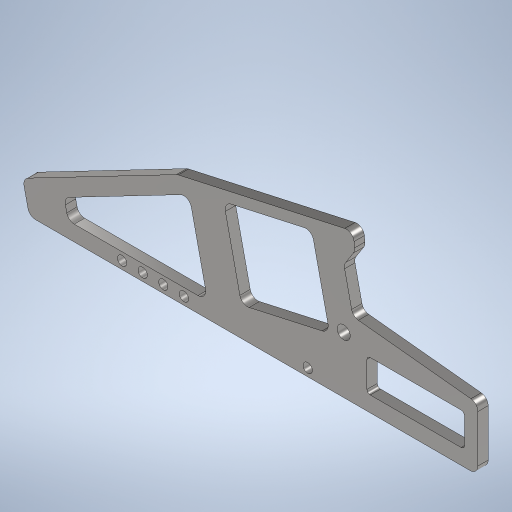
# Autodesk Inventor part: Uprights
Saved by Autodesk Inventor 2023.4 (Build 274418000, 418)
## iProperties
Created: 2024-02-11
Part Number: Uprights
Material: Stainless Steel
Document SubType Name: Modeling
Designer: Nathan Cai
Density: 8 g/cm^3
Appearance: Semi-Polished
Mass: 70.807 g
Surface Area: 79.2126 cm^2
Volume: 8.85087 cm^3
Author: Nathan Cai
Autodesk Inventor part; units mm, degrees
ref_plane "YZ Plane" through (0, 0, 0) normal (1, 0, 0) x (0, 1, 0)
ref_plane "XZ Plane" through (0, 0, 0) normal (0, 1, 0) x (-1, 0, 0)
ref_plane "XY Plane" through (0, 0, 0) normal (0, 0, 1) x (1, 0, 0)
sketch "Sketch1" plane through (0, 0, 0) normal (0, 0, 1) x (1, 0, 0)
  line L0 (0, 0) -> (0, 136.2362)
  line L1 (-14.9636, 12.2907) -> (-39.7615, 17.7883)
  line L2 (-39.7615, 17.7883) -> (-33.7485, 44.911)
  line L3 (-33.7485, 44.911) -> (-8.9506, 39.4135)
  line L4 (-8.9506, 39.4135) -> (-14.9636, 12.2907)
  line L5 (-39.7615, 17.7883) -> (-8.9506, 39.4135) construction
  line L6 (-33.7485, 44.911) -> (-14.9636, 12.2907) construction
  circle A0 centre (-57.15, 12.7) radius 3.3401
  circle A1 centre (-57.15, 12.7) radius 6.35
  line L7 (0, 0) -> (-57.847, 6.3884)
  line L8 (-62.7825, 15.6321) -> (0, 136.2362)
  line L9 (-21.3496, 42.1622) -> (-27.3626, 15.0395) construction
  line L10 (0, 104.775) -> (-14.6831, 108.0302)
  line L11 (-35.4518, 7.8896) -> (-23.0529, 5.1408)
  line L12 (-23.0529, 5.1408) -> (-24.4273, -1.0586) construction
  line L13 (-24.4273, -1.0586) -> (-36.8262, 1.6901) construction
  line L14 (-36.8262, 1.6901) -> (-35.4518, 7.8896) construction
  line L15 (-35.4518, 7.8896) -> (-40.7688, 4.5023)
  line L16 (-8.9506, 39.4135) -> (-33.7485, 44.911)
  line L17 (-56.4271, 15.9609) -> (-57.15, 12.7) construction
  line L18 (-57.15, 12.7) -> (-60.4109, 13.4229) construction
  line L19 (-29.2523, 6.5152) -> (-36.1243, -24.4822) construction
  line L20 (-56.356, 15.9443) -> (-9.0672, 106.7852)
  line L21 (-35.1857, 56.612) -> (0, 48.8115)
  line L22 (-4.7625, 49.8673) -> (-4.7625, 105.8308)
  line L23 (-30.3721, 55.5448) -> (-10.3247, 94.0556)
  line L24 (-10.3247, 94.0556) -> (-4.7625, 92.8225)
  circle A2 centre (-17.3978, 7.9523) radius 2
  line L25 (0, 13.4938) -> (-4.7625, 13.4937) construction
  line L26 (-4.7625, 13.4937) -> (-4.7625, 24.6063) construction
  line L27 (-4.7625, 24.6063) -> (0, 24.6063) construction
  line L28 (0, 24.6063) -> (0, 13.4938) construction
  line L29 (-4.7625, 19.05) -> (0, 19.05) construction
  circle A3 centre (-2.3812, 19.05) radius 1.4224
  line L30 (-4.7625, 57.15) -> (0, 57.15) construction
  circle A4 centre (-2.3813, 57.15) radius 1.4224
  circle A5 centre (-2.3813, 63.5) radius 1.4224
  circle A6 centre (-2.3813, 69.85) radius 1.4224
  circle A7 centre (-2.3813, 76.2) radius 1.4224
  line L31 (-22.792, 92.4532) -> (-17.8635, 89.8876)
  circle A8 centre (-57.15, 12.7) radius 9.525 construction
  line L32 (-14.7625, 0.7937) -> (-4.7625, 0.7938)
  line L33 (-4.7625, 0.7938) -> (-4.7625, -29.2062)
  line L34 (-4.7625, -29.2062) -> (-14.7625, -29.2062)
  line L35 (-14.7625, -29.2062) -> (-14.7625, 0.7937)
  line L36 (-14.7625, 0.7937) -> (-4.7625, -29.2062) construction
  line L37 (-4.7625, 0.7938) -> (-14.7625, -29.2062) construction
  line L38 (-19.05, -33.3375) -> (0, -33.3375)
  line L39 (0, -33.3375) -> (0, 0)
  line L40 (-23.0529, 5.1408) -> (-19.05, -33.3375)
  circle A9 centre (-17.3978, 7.9523) radius 6.5 construction
  line L41 (-22.7129, 14.0087) -> (-24.6027, 5.4844) construction
  line L42 (-17.3978, 7.9523) -> (-23.8273, 9.3776) construction
  line L43 (-33.8287, 59.2189) -> (-45.835, 5.0618)
  point P0 (-24.3561, 28.6009)
  point P1 (-23.6144, 2.6079)
  point P2 (-36.3119, 4.0101)
  point P3 (-54.945, 18.6549)
  point P4 (0, 48.8115)
  point P5 (-24.3561, 28.6009)
  point P6 (-9.7625, -14.2062)
  dimension "d14" = 27.7812
  dimension "d15" = 25.4
  dimension "d16" = 12.5
  dimension "d17" = 6.6802
  dimension "d19" = 57.15
  dimension "d22" = 12.7
  dimension "d26" = 102.5
  dimension "d29" = 6.35
  dimension "d31" = 6.35
  dimension "d35" = 28.575
  dimension "d38" = 31.75
  dimension "d55" = 4.7625
  dimension "d56" = 4.7625
  dimension "d60" = 12.7
  dimension "d66" = 4
  dimension "d72" = 8.7312
  dimension "d80" = 104.775
  dimension "d85" = 4.7625
  dimension "d86" = 11.1125
  dimension "d87" = 2.8448
  dimension "d88" = 19.05
  dimension "d89" = 2.8448
  dimension "d90" = 38.1
  dimension "d93" = 6.35
  dimension "d104" = 27.5
  dimension "d105" = 5.5563
  dimension "d106" = 19.05
  dimension "d111" = 19.05
  dimension "d112" = 10
  dimension "d113" = 30
  dimension "d114" = 4.7625
  dimension "d115" = 0.7937
  dimension "d117" = 19.05
  dimension "d119" = 11.1125
  dimension "d120" = 12.7
  dimension "d121" = 33.3375
  dimension "d122" = 45
  dimension "d123" = 13
  dimension "d124" = 4.7625
  dimension "d125" = 4.7625
  dimension "d126" = 3.175
  constraints: 88 end point, 20 point on line, 14 parallel, 11 midpoint, 11 perpendicular, 10 centre point, 9 coincident, 5 point on circle, 3 horizontal, 3 tangent, 3 vertical, 1 collinear, 7 other
  measures "d14" distance of L1.end L2.end
  measures "d15" distance between parallel lines of L4 L2
  measures "d16" angle of L0 L4
  measures "d17" diameter of A0
  measures "d19" distance from line of L0 A0.centre
  measures "d22" diameter of A1
  measures "d26" angle of L0 L10
  measures "d29" distance of L11.end L12.end
  measures "d31" distance between parallel lines of L12 L9
  measures "d35" distance between parallel lines of L9 L17
  measures "d38" distance of L19.start L19.end
  measures "d55" distance between parallel lines of L0 L22
  measures "d56" distance between parallel lines of L20 L23
  measures "d60" vertical distance of A0.centre L0.start
  measures "d66" diameter of A2
  measures "d72" distance between parallel lines of L1 L11
  measures "d80" distance of L0.start point (0, 104.775)
  measures "d85" distance of L26.end L27.end
  measures "d86" distance between parallel lines of L25 L27
  measures "d87" diameter of A3
  measures "d88" distance from line of L39.end L29
  measures "d89" diameter of A4
  measures "d90" distance between parallel lines of L29 L30
  measures "d93" distance of A4.centre A5.centre
  measures "d104" angle of L0 L8
  measures "d105" distance between parallel lines of L8 L20
  measures "d106" distance from line of L20.end L31
  measures "d111" diameter of A8
  measures "d112" distance of L33.end L34.end
  measures "d113" distance of L32.end L33.end
  measures "d114" distance between parallel lines of L0 L33
  measures "d115" distance from line of L0.start L32
  measures "d117" distance of L38.start L38.end
  measures "d119" distance between parallel lines of L16 L21
  measures "d120" distance between parallel lines of L10 L24
  measures "d121" distance from line of L38 L0.start
  measures "d122" angle of L15 L14
  measures "d123" diameter of A9
  measures "d124" distance between parallel lines of L9 L41
  measures "d125" distance between parallel lines of L1 L42
  measures "d126" distance between parallel lines of L2 L43
extrude "Extrusion1" add sketch "Sketch1" along normal blind 3.175 contours L7 L33 L32 L40 L11 L15 L43 L21 L0 | L39 L38 L40 L7 L32 L35 L34 L33 | L21 L22 L10 L0 | L22 L24 L23 L21 L43 L20 L10
fillet "Fillet1" radius 2.3813 17 edges at (-39.7615, 17.7883, 1.5875) (-14.9636, 12.2907, 1.5875) (-23.0529, 5.1408, 1.5875) (-35.4518, 7.8896, 1.5875) (-40.7688, 4.5023, 1.5875) (-4.7625, 92.8225, 1.5875) (-30.3721, 55.5448, 1.5875) (-4.7625, 49.8673, 1.5875) (-33.7485, 44.911, 1.5875) (-8.9506, 39.4135, 1.5875) (-19.05, -33.3375, 1.5875) (0, -33.3375, 1.5875) (-10.3247, 94.0556, 1.5875) (-33.8287, 59.2189, 1.5875) (-45.835, 5.0618, 1.5875) (-9.0672, 106.7852, 1.5875) (0, 104.775, 1.5875)
fillet "Fillet6" radius 1 4 edges at (-4.7625, 0.7938, 1.5875) (-14.7625, 0.7937, 1.5875) (-14.7625, -29.2062, 1.5875) (-4.7625, -29.2062, 1.5875)
equation "\"d56\" = d55"
body "Solid1"
